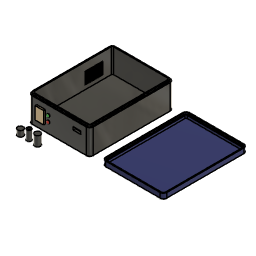
Caixa_IEB v5 (Autodesk Fusion 360 design; units mm, degrees)
Autodesk Fusion 360 part; units mm, degrees
sketch "Sketch1" plane through (0, 0, 0) normal (0, 0, 1) x (1, 0, 0)
  line L0 (2, 0) -> (98, 0)
  line L1 (100, -2) -> (100, -138)
  line L2 (98, -140) -> (2, -140)
  line L3 (0, -138) -> (0, -2)
  arc A0 (2, 0) -> (0, -2) centre (2, -2) ccw
  arc A1 (100, -2) -> (98, 0) centre (98, -2) ccw
  arc A2 (98, -140) -> (100, -138) centre (98, -138) ccw
  arc A3 (0, -138) -> (2, -140) centre (2, -138) ccw
  arc A4 (102, -2) -> (98, 2) centre (98, -2) ccw
  line L4 (2, 2) -> (98, 2)
  arc A5 (2, 2) -> (-2, -2) centre (2, -2) ccw
  line L5 (-2, -138) -> (-2, -2)
  arc A6 (-2, -138) -> (2, -142) centre (2, -138) ccw
  line L6 (98, -142) -> (2, -142)
  arc A7 (98, -142) -> (102, -138) centre (98, -138) ccw
  line L7 (102, -2) -> (102, -138)
  arc A8 (104, -2) -> (98, 4) centre (98, -2) ccw
  line L8 (2, 4) -> (98, 4)
  arc A9 (2, 4) -> (-4, -2) centre (2, -2) ccw
  line L9 (-4, -138) -> (-4, -2)
  arc A10 (-4, -138) -> (2, -144) centre (2, -138) ccw
  line L10 (98, -144) -> (2, -144)
  arc A11 (98, -144) -> (104, -138) centre (98, -138) ccw
  line L11 (104, -2) -> (104, -138)
  arc A12 (102.2, -2) -> (98, 2.2) centre (98, -2) ccw
  line L12 (2, 2.2) -> (98, 2.2)
  arc A13 (2, 2.2) -> (-2.2, -2) centre (2, -2) ccw
  line L13 (-2.2, -138) -> (-2.2, -2)
  arc A14 (-2.2, -138) -> (2, -142.2) centre (2, -138) ccw
  line L14 (98, -142.2) -> (2, -142.2)
  arc A15 (98, -142.2) -> (102.2, -138) centre (98, -138) ccw
  line L15 (102.2, -2) -> (102.2, -138)
  point P0 (100, 0)
  point P1 (0, -140)
  dimension "d1" = 140
  dimension "d2" = 100
  dimension "d3" = 2
  dimension "d4" = -2
  dimension "d5" = -4
  dimension "d6" = -2.2
  constraint horizontal L0
  constraint vertical L1
  constraint horizontal L2
  constraint vertical L3
  constraint coincident origin L0
  constraint coincident origin L3
  constraint tangent L0 A0
  constraint tangent L3 A0
  constraint coincident P0 L0
  constraint coincident P0 L1
  constraint tangent L0 A1
  constraint tangent L1 A1
  constraint equal A0 A1
  constraint tangent L1 A2
  constraint tangent L2 A2
  constraint equal A0 A2
  constraint coincident P1 L2
  constraint coincident P1 L3
  constraint tangent L2 A3
  constraint tangent L3 A3
  constraint equal A0 A3
  measures "d1" distance of origin P1
  measures "d2" distance of origin P0
  measures "d3" radius of A0
  measures "d4" distance of A1
  measures "d5" distance of A1
extrude "Extrude1" add sketch "Sketch1" against normal blind 5 contours L0 L1 L2 L3 A0 A1 A2 A3 | A4 L4 A5 L5 A6 L6 A7 L7 | A8 L8 A9 L9 A10 L10 A11 L11 | A12 L12 A13 L13 A14 L14 A15 L15 makes body 1
extrude "Extrude2" add sketch "Sketch1" along normal blind 42.5 contours A4 L4 A5 L5 A6 L6 A7 L7 bodies 1
extrude "Extrude3" add sketch "Sketch1" along normal up to surface (40 mm away) contours A8 L8 A9 L9 A10 L10 A11 L11 | A12 L12 A13 L13 A14 L14 A15 L15 bodies 1
copy_body "Body->Comp1" bodies 1 removing the originals makes body 2 in component "Component"
extrude "Extrude1'" add sketch "Sketch1" along normal blind 10 from surface at 40 separate body contours A8 L8 A9 L9 A10 L10 A11 L11 makes body 3 in component "Component'"
extrude "Extrude2'" add sketch "Sketch1" against normal blind 7.5 from surface at 50 contours A4 L4 A5 L5 A6 L6 A7 L7 | A12 L12 A13 L13 A14 L14 A15 L15 bodies 3 in component "Component'"
extrude "Extrude3'" add sketch "Sketch1" against normal blind 3 from surface at 50 contours L0 L1 L2 L3 A0 A1 A2 A3 bodies 3 in component "Component'"
fillet "Fillet1" radius 1.5 8 edges at (50, -144, -5) (-2.2426, -142.2426, -5) (-4, -70, -5) (-2.2426, 2.2426, -5) (50, 4, -5) (102.2426, 2.2426, -5) (104, -70, -5) (102.2426, -142.2426, -5) on bodies 2 in component "Component"
fillet "Fillet1'" radius 1.5 8 edges at (50, 4, 50) (-2.2426, 2.2426, 50) (-4, -70, 50) (-2.2426, -142.2426, 50) (50, -144, 50) (102.2426, -142.2426, 50) (104, -70, 50) (102.2426, 2.2426, 50) on bodies 3 in component "Component'"
sketch "Sketch2" plane through (0, -144, 0) normal (0, -1, 0) x (1, 0, 0)
  line L0 (2, -3.5) -> (98, -3.5)
  line L1 (98, -3.5) -> (98, 40)
  line L2 (98, 40) -> (2, 40)
  line L3 (2, 40) -> (2, -3.5)
  line L4 (12, 29) -> (24.2, 29)
  line L5 (24.2, 29) -> (24.2, 10)
  line L6 (24.2, 10) -> (12, 10)
  line L7 (12, 10) -> (12, 29)
  line L8 (0, 0) -> (0, 42.5)
  line L9 (0, 42.5) -> (0, 0)
  line L10 (2, -5) -> (98, -5)
  line L11 (74.7, 29) -> (88, 29)
  line L12 (88, 29) -> (88, 23.8)
  line L13 (88, 23.8) -> (74.7, 23.8)
  line L14 (74.7, 23.8) -> (74.7, 29)
  line L15 (74.7, 29) -> (24.2, 29) construction
  line L16 (100, 0) -> (100, 42.5) construction
  line L17 (100, 42.5) -> (100, 0) construction
  line L18 (24.2, 19.5) -> (31.2, 19.5) construction
  line L19 (31.2, 19.5) -> (31.2, 24.5) construction
  line L20 (31.2, 19.5) -> (31.2, 14.5) construction
  circle A0 centre (31.2, 24.5) radius 2.5
  circle A1 centre (31.2, 14.5) radius 2.5
  dimension "d27" = 12.2
  dimension "d28" = 19
  dimension "d29" = 12
  dimension "d30" = 15
  dimension "d31" = 5.2
  dimension "d32" = 13.3
  dimension "d45" = 11
  dimension "d47" = 12
  dimension "d78" = 5
  dimension "d79" = 10
  dimension "d80" = 7
  constraint horizontal L4
  constraint vertical L5
  constraint horizontal L6
  constraint vertical L7
  constraint horizontal L11
  constraint vertical L12
  constraint horizontal L13
  constraint vertical L14
  constraint horizontal L15
  constraint midpoint L5 L18.start
  constraint perpendicular L5 L18
  constraint perpendicular L18 L19
  constraint perpendicular L18 L20
  constraint equal L19 L20
  constraint coincident L19.end A0.centre
  constraint coincident L20.end A1.centre
  constraint equal A0 A1
  measures "d27" distance of L4.start L4.end
  measures "d28" distance of L4.start L6.end
  measures "d29" distance of L7 L9
  measures "d30" distance of L6 L10
  measures "d31" distance of L11.start L13.end
  measures "d32" distance of L11.start L11.end
  measures "d45" distance of L2 L4
  measures "d47" distance of L12 L16
  measures "d78" diameter of A0
  measures "d79" distance of L19.end L20.end
  measures "d80" distance of L18.start L18.end
extrude "Extrude1''" cut sketch "Sketch2" against normal blind 20 contours L4 L5 L6 L7 | L11 L12 L13 L14 | A0 | A1 bodies 2 in component "Component"
sketch "Sketch3" plane through (0, 0, 0) normal (0, 0, 1) x (-1, 0, 0)
  line L0 (0, 2) -> (0, 138)
  arc A0 (0, 138) -> (-2, 140) centre (-2, 138) ccw
  line L1 (-2, 140) -> (-98, 140)
  arc A1 (-98, 140) -> (-100, 138) centre (-98, 138) ccw
  line L2 (-100, 138) -> (-100, 2)
  arc A2 (-100, 2) -> (-98, 0) centre (-98, 2) ccw
  line L3 (-98, 0) -> (-2, 0)
  arc A3 (-2, 0) -> (0, 2) centre (-2, 2) ccw
  circle A4 centre (-71, 13) radius 4
  circle A5 centre (-71, 13) radius 2
  line L4 (-71, 13) -> (-71, 131) construction
  circle A6 centre (-71, 131) radius 4
  circle A7 centre (-71, 131) radius 2
  dimension "d36" = 8
  dimension "d37" = 4
  dimension "d38" = 118
  dimension "d39" = 29
  dimension "d40" = 13
  constraint concentric A4 A5
  constraint coincident A4.centre A5.centre
  constraint vertical L4
  constraint coincident L4.end A6.centre
  constraint equal A4 A6
  constraint equal A5 A7
  measures "d36" diameter of A4
  measures "d37" diameter of A5
  measures "d38" distance of A4.centre L4.end
  measures "d39" distance of L2 L4
  measures "d40" distance of L3 A4.centre
extrude "Extrude2''" cut sketch "Sketch3" against normal blind 25 contours A5 | A7 bodies 2 in component "Component"
extrude "Extrude3''" cut sketch "Sketch3" against normal blind 2.5 contours A4 | A6 bodies 2 in component "Component"
sketch "Sketch4" plane through (0, 0, 0) normal (0, 0, 1) x (1, 0, 0)
  circle A0 centre (12, -174) radius 5
  line L0 (12, -174) -> (27, -174) construction
  line L1 (27, -174) -> (42, -174) construction
  circle A1 centre (27, -174) radius 4
  circle A2 centre (27, -174) radius 2
  circle A3 centre (42, -174) radius 5
  line L2 (98, -144) -> (2, -144)
  dimension "d48" = 10
  dimension "d49" = 15
  dimension "d50" = 15
  dimension "d51" = 8
  dimension "d52" = 4
  dimension "d53" = 10
  dimension "d62" = 30
  dimension "d63" = 10
  constraint coincident A0.centre L0.start
  constraint horizontal L0
  constraint parallel L0 L1
  constraint coincident L0.end L1.start
  constraint coincident L1.end A3.centre
  measures "d48" diameter of A0
  measures "d49" distance of A0.centre L0.end
  measures "d50" distance of L0.end L1.end
  measures "d51" diameter of A1
  measures "d52" diameter of A2
  measures "d53" diameter of A3
  measures "d62" distance of L0 L2
  measures "d63" horizontal distance of A0.centre L2.end
extrude "Extrude4" add sketch "Sketch4" along normal blind 17.2 separate body contours A3 makes body 4
extrude "Extrude5" add sketch "Sketch4" along normal blind 3 separate body contours A2 makes body 5
extrude "Extrude6" add sketch "Sketch4" along normal blind 17 contours A1 bodies 5
extrude "Extrude7" add sketch "Sketch4" along normal blind 10 separate body contours A0 makes body 6
sketch "Sketch5" plane through (0, 0, -5) normal (0, 0, -1) x (1, 0, 0)
  circle A0 centre (71, 13) radius 2
  circle A1 centre (71, 131) radius 2
  line L0 (98, 142.5) -> (2, 142.5)
  arc A2 (2, 142.5) -> (-2.5, 138) centre (2, 138) ccw
  line L1 (-2.5, 138) -> (-2.5, 2)
  arc A3 (-2.5, 2) -> (2, -2.5) centre (2, 2) ccw
  line L2 (2, -2.5) -> (98, -2.5)
  arc A4 (98, -2.5) -> (102.5, 2) centre (98, 2) ccw
  line L3 (102.5, 2) -> (102.5, 138)
  arc A5 (102.5, 138) -> (98, 142.5) centre (98, 138) ccw
  line L4 (7.5, 132.5) -> (7.5, 7.5) construction
  line L5 (7.5, 7.5) -> (92.5, 7.5) construction
  line L6 (92.5, 7.5) -> (92.5, 132.5) construction
  line L7 (92.5, 132.5) -> (7.5, 132.5) construction
  circle A6 centre (7.5, 132.5) radius 5.15
  circle A7 centre (92.5, 132.5) radius 5.15
  circle A8 centre (92.5, 7.5) radius 5.15
  circle A9 centre (7.5, 7.5) radius 5.15
  point P0 (50, 70)
  dimension "d64" = -10
  dimension "d65" = 10.3
  constraint coincident L4.start L7.end
  constraint coincident L6.end L7.start
  constraint coincident L5.end L6.start
  constraint coincident L4.end L5.start
  constraint equal A6 A7
  constraint equal A6 A9
  constraint equal A6 A8
  measures "d65" diameter of A6
extrude "Extrude4'" cut sketch "Sketch5" against normal blind 0.6 contours A6 | A7 | A8 | A9 bodies 2 in component "Component"
sketch "Sketch6" plane through (-4, 0, 0) normal (-1, 0, 0) x (0, -1, 0)
  line L0 (2, -3.5) -> (138, -3.5)
  line L1 (138, -3.5) -> (138, 40)
  line L2 (138, 40) -> (2, 40)
  line L3 (2, 40) -> (2, -3.5)
  line L4 (17, 28) -> (18, 28)
  line L5 (18, 28) -> (18, 7)
  line L6 (18, 7) -> (17, 7)
  line L7 (17, 7) -> (17, 28)
  line L8 (-4, 40) -> (-4, -3.5)
  line L9 (20, 28) -> (20, 7)
  line L10 (20, 7) -> (19, 7)
  line L11 (19, 28) -> (20, 28)
  line L12 (19, 7) -> (19, 28)
  line L13 (22, 28) -> (22, 7)
  line L14 (22, 7) -> (21, 7)
  line L15 (21, 28) -> (22, 28)
  line L16 (21, 7) -> (21, 28)
  line L17 (24, 28) -> (24, 7)
  line L18 (24, 7) -> (23, 7)
  line L19 (23, 28) -> (24, 28)
  line L20 (23, 7) -> (23, 28)
  line L21 (26, 28) -> (26, 7)
  line L22 (26, 7) -> (25, 7)
  line L23 (25, 28) -> (26, 28)
  line L24 (25, 7) -> (25, 28)
  line L25 (28, 28) -> (28, 7)
  line L26 (28, 7) -> (27, 7)
  line L27 (27, 28) -> (28, 28)
  line L28 (27, 7) -> (27, 28)
  line L29 (30, 28) -> (30, 7)
  line L30 (30, 7) -> (29, 7)
  line L31 (29, 28) -> (30, 28)
  line L32 (29, 7) -> (29, 28)
  line L33 (32, 28) -> (32, 7)
  line L34 (32, 7) -> (31, 7)
  line L35 (31, 28) -> (32, 28)
  line L36 (31, 7) -> (31, 28)
  line L37 (34, 28) -> (34, 7)
  line L38 (34, 7) -> (33, 7)
  line L39 (33, 28) -> (34, 28)
  line L40 (33, 7) -> (33, 28)
  line L41 (36, 28) -> (36, 7)
  line L42 (36, 7) -> (35, 7)
  line L43 (35, 28) -> (36, 28)
  line L44 (35, 7) -> (35, 28)
  line L45 (38, 28) -> (38, 7)
  line L46 (38, 7) -> (37, 7)
  line L47 (37, 28) -> (38, 28)
  line L48 (37, 7) -> (37, 28)
  line L49 (40, 28) -> (40, 7)
  line L50 (40, 7) -> (39, 7)
  line L51 (39, 28) -> (40, 28)
  line L52 (39, 7) -> (39, 28)
  line L53 (42, 28) -> (42, 7)
  line L54 (42, 7) -> (41, 7)
  line L55 (41, 28) -> (42, 28)
  line L56 (41, 7) -> (41, 28)
  line L57 (44, 28) -> (44, 7)
  line L58 (44, 7) -> (43, 7)
  line L59 (43, 28) -> (44, 28)
  line L60 (43, 7) -> (43, 28)
  line L61 (46, 28) -> (46, 7)
  line L62 (46, 7) -> (45, 7)
  line L63 (45, 28) -> (46, 28)
  line L64 (45, 7) -> (45, 28)
  line L65 (48, 28) -> (48, 7)
  line L66 (48, 7) -> (47, 7)
  line L67 (47, 28) -> (48, 28)
  line L68 (47, 7) -> (47, 28)
  dimension "d68" = 12
  dimension "d69" = 21
  dimension "d70" = 1
  dimension "d71" = 21
  dimension "d74" = 2
  dimension "d75" = 0
  constraint horizontal L4
  constraint vertical L5
  constraint horizontal L6
  constraint vertical L7
  measures "d68" distance of L2 L4
  measures "d69" distance of L7 L8
  measures "d70" distance of L5 L7
  measures "d71" distance of L4.start L6.end
extrude "Extrude5'" cut sketch "Sketch6" against normal blind 10 contours L4 L5 L6 L7 | L9 L10 L11 L12 | L13 L14 L15 L16 | L17 L18 L19 L20 | L21 L22 L23 L24 | L25 L26 L27 L28 | L29 L30 L31 L32 | L33 L34 L35 L36 | L37 L38 L39 L40 | L41 L42 L43 L44 | L45 L46 L47 L48 | L49 L50 L51 L52 | L53 L54 L55 L56 | L57 L58 L59 L60 | L61 L62 L63 L64 | L65 L66 L67 L68 bodies 2 in component "Component"
move_body "Move1" bodies 3 to x (-1, 0, 0) y (0, 1, 0) z (0, 0, -1) at (230, 0, 45) in component "Component'"
sketch "Sketch7" plane through (0, -144, 0) normal (0, -1, 0) x (1, 0, 0)
  line L0 (88, 29) -> (88, 23.8)
  line L1 (88, 23.8) -> (74.7, 23.8)
  line L2 (74.7, 23.8) -> (74.7, 29)
  line L3 (74.7, 29) -> (88, 29)
  circle A0 centre (31.2, 24.5) radius 2.5
  line L4 (24.2, 29) -> (24.2, 10)
  line L5 (24.2, 10) -> (12, 10)
  line L6 (12, 10) -> (12, 29)
  line L7 (12, 29) -> (24.2, 29)
  circle A1 centre (31.2, 14.5) radius 2.5
  line L8 (2, -3.5) -> (98, -3.5)
  line L9 (98, -3.5) -> (98, 40)
  line L10 (98, 40) -> (2, 40)
  line L11 (2, 40) -> (2, -3.5)
  line L12 (25.7, 8.5) -> (10.5, 8.5)
  line L13 (10.5, 8.5) -> (10.5, 30.5)
  line L14 (10.5, 30.5) -> (25.7, 30.5)
  line L15 (25.7, 30.5) -> (25.7, 8.5)
  dimension "d81" = -1.5
extrude "Extrude1'''" add sketch "Sketch7" along normal blind 3 separate body contours A0 | L4 L5 L6 L7 | A1 | L12 L13 L14 L15 makes body 7 at (33.6876, -145, 24.2511) makes body 8 at (33.6876, -145, 14.2511) makes body 9 at (20.6333, -144, 15.8333) in component "Component''"
fillet "Fillet1''" radius 2.5 2 edges at (28.8692, -147, 23.596) (28.8692, -147, 13.596) on bodies 7 8 in component "Component''"
component "Component" placed x (1, 0, 0) y (0, 1, 0) z (0, 0, 1) at (0, 0, 0)
component "Component'" placed x (1, 0, 0) y (0, 1, 0) z (0, 0, 1) at (0, 0, 0)
component "Component''" placed x (1, 0, 0) y (0, 1, 0) z (0, 0, 1) at (0, 0, 0)
named bodies: "Base"
